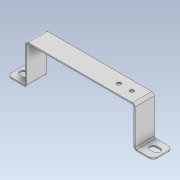
# Autodesk Inventor part: Скоба БП2
Saved by Autodesk Inventor 2021.2 (Build 252289000, 289)
## iProperties
Created: 2022-11-30
Part Number: Скоба БП2
Material: Типовые
Document SubType Name: ЛистМат
Designer: Voodoo
Mass: 2.46524 g
Surface Area: 53.5844 cm^2
Volume: 2.46524 cm^3
Density: 1 g/cm^3
Sheet Metal Rule: По умолчанию_мм
Appearance: По умолчанию
Author: Voodoo
Autodesk Inventor part; units mm, degrees
ref_plane "YZ Plane" through (0, 0, 0) normal (1, 0, 0) x (0, 1, 0)
ref_plane "XZ Plane" through (0, 0, 0) normal (0, 1, 0) x (-1, 0, 0)
ref_plane "XY Plane" through (0, 0, 0) normal (0, 0, 1) x (1, 0, 0)
sketch "Эскиз1" plane through (0, 0, 0) normal (0, 0, 1) x (1, 0, 0)
  line L0 (0, 0) -> (83, 0) construction
  line L1 (83, 0) -> (83, 30)
  line L2 (83, 30) -> (0, 30)
  line L3 (0, 30) -> (0, 0)
  line L4 (0, 0) -> (-15, 0)
  line L5 (83, 0) -> (98, 0)
  dimension "d0" = 83
  dimension "d1" = 30
  dimension "d2" = 15
  dimension "d3" = 15
  measures "d0" distance of L1.end L2.end
  measures "d1" distance between parallel lines of L0 L2
  measures "d2" distance of L0.start L4.end
  measures "d3" distance of L0.end L5.end
contour flange "Фланец по контуру1" sketch "Эскиз1" thickness 1 bend radius 1 width 15 along (0, 0, 1) mid plane no both sides no wall seen from (-7.5, 0, 0) lies toward (0, 1, 0) curves L4 L3 L2 L1 L5
bend "Сгиб1"
corner "УглСтык1"
sketch "Эскиз2" plane through (98, 1, 15) normal (0, 1, 0) x (1, 0, 0)
  line L0 (-100, 15) -> (-100, 0) projected
  line L1 (-113, 15) -> (-100, 15) projected
  line L2 (-113, 0) -> (-113, 15) projected
  line L3 (-100, 0) -> (-113, 0) projected
  line L4 (-13, 15) -> (-13, 0) projected
  line L5 (0, 0) -> (-13, 0) projected
  line L6 (0, 15) -> (0, 0) projected
  line L7 (-13, 15) -> (0, 15) projected
  line L8 (-7.5, 7.5) -> (-4.5, 7.5) construction
  line L9 (-7.5, 5) -> (-4.5, 5)
  line L10 (-4.5, 10) -> (-7.5, 10)
  arc A0 (-7.5, 10) -> (-7.5, 5) centre (-7.5, 7.5) ccw
  arc A1 (-4.5, 5) -> (-4.5, 10) centre (-4.5, 7.5) ccw
  line L11 (-108.5, 7.5) -> (-105.5, 7.5) construction
  line L12 (-108.5, 5) -> (-105.5, 5)
  line L13 (-105.5, 10) -> (-108.5, 10)
  arc A2 (-108.5, 10) -> (-108.5, 5) centre (-108.5, 7.5) ccw
  arc A3 (-105.5, 5) -> (-105.5, 10) centre (-105.5, 7.5) ccw
  point P0 (-98, 15)
  point P1 (-6, 7.5)
  point P2 (-107, 7.5)
  point P3 (-113, 7.5)
  point P4 (0, 7.5)
  dimension "d15" = 3
  dimension "d16" = 5
  dimension "d17" = 3
  dimension "d18" = 5
  dimension "d19" = 6
  dimension "d20" = 6
  constraints: 16 end point, 8 point on circle, 8 tangent, 4 centre point, 4 midpoint, 2 horizontal, 2 horizontal alignment, 2 parallel
  measures "d15" distance of L8.start L8.end
  measures "d16" diameter of A1
  measures "d17" distance of L11.start L11.end
  measures "d18" diameter of A3
  measures "d19" distance from line of L6 point (-6, 7.5)
  measures "d20" distance from line of L2 point (-107, 7.5)
extrude "Вырез1" cut sketch "Эскиз2" against normal blind 1 contours A0 L10 A1 L9 | A2 L13 A3 L12
fillet "УглСкругление1" radius 3 4 edges at (-15, 0.5, 15) (-15, 0.5, 0) (98, 0.5, 15) (98, 0.5, 0)
sketch "Эскиз3" plane through (1, 31, 0) normal (0, 1, 0) x (1, 0, 0)
  line L0 (81, 0) -> (81, -15) projected
  line L1 (0, 0) -> (81, 0) projected
  line L2 (0, 0) -> (0, -15) projected
  line L3 (81, -15) -> (0, -15) projected
  circle A0 centre (73, -7.5) radius 1.5
  circle A1 centre (63, -7.5) radius 1.5
  point P0 (-1, 0)
  point P1 (81, -7.5)
  dimension "d24" = 3
  dimension "d25" = 8
  dimension "d28" = 3
  dimension "d29" = 10
  constraints: 2 centre point, 2 horizontal alignment, 1 midpoint
  measures "d24" diameter of A0
  measures "d25" distance from line of A0.centre L0
  measures "d28" diameter of A1
  measures "d29" distance of A0.centre A1.centre
extrude "Вырез2" cut sketch "Эскиз3" against normal blind 1 contours A0 | A1
equation "\"d21\" = Толщина"
equation "\"d26\" = Толщина"
equation "\"d4\" = Толщина"
equation "\"d5\" = Ширина_просечки"
equation "\"d6\" = Глубина_просечки"
equation "\"d7\" = Мин_остаток"
equation "\"d8\" = Радиус_перехода"
equation "\"d10\" = Радиус_гибки"
equation "\"d12\" = Размер_просечки"
equation "\"d13\" = Размер_зазора"
equation "\"d14\" = Радиус_Якоби"
equation "\"Радиус_гибки\" = Толщина"
equation "\"Ширина_просечки\" = Толщина"
equation "\"Глубина_просечки\" = 0.5 * Толщина"
equation "\"Размер_просечки\" = 4 * Толщина"
equation "\"Мин_остаток\" = 2 * Толщина"
equation "\"Радиус_перехода\" = Радиус_гибки"
equation "\"Радиус_Якоби\" = Радиус_гибки"
equation "\"Размер_зазора\" = Толщина"
equation "\"Толщина\" = 1"
